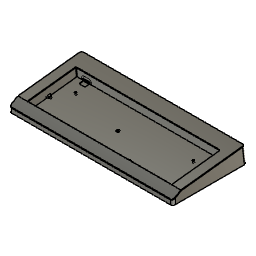
Bezel (Autodesk Fusion 360 design; units mm, degrees)
Autodesk Fusion 360 part; units mm, degrees
note: some values were not read from the file. Set by a fixed rule: which sketch regions a step uses.
sketch "スケッチ1" plane through (0, 0, 0) normal (1, 0, 0) x (0, 1, 0)
  line L0 (17.006428, 19.886797) -> (113.581613, 30.890149)
  line L1 (20.037658, 2.115707) -> (115.61927, 13.005856)
  line L2 (115.61927, 13.005856) -> (113.581613, 30.890149)
  line L3 (20.037658, 2.115707) -> (0.037658, 2.115707)
  line L4 (0.037658, 2.115707) -> (0.037658, 10.089873)
  line L5 (0.037658, 10.089873) -> (17.006428, 19.886797)
  line L6 (113.581613, 30.890149) -> (144.38234, 34.399449)
  line L7 (144.38234, 34.399449) -> (146.419998, 16.515155)
  line L8 (146.419998, 16.515155) -> (139.289315, 0.115707)
  line L9 (0.037658, 2.115707) -> (0.037658, 0.115707)
  line L10 (0.037658, 0.115707) -> (139.000002, 0.115707)
  line L11 (139.000002, 0.115707) -> (139.289315, 0.115707)
  line L12 (115.61927, 13.005856) -> (146.419998, 16.515155)
  line L13 (139.289315, 0.115707) -> (149.000002, 0.115707)
  line L14 (146.419998, 16.515155) -> (148.288479, 0.115707)
  line L15 (0.037658, 10.089873) -> (-9.962342, 4.31637)
  line L16 (0.037658, 0.115707) -> (-9.962342, 0.115707)
  line L17 (-9.962342, 0.115707) -> (-9.962342, 4.31637)
  dimension "d5" = 90
  dimension "d6" = 20
  dimension "d7" = 31
  dimension "d8" = 150
  dimension "d9" = 2
  dimension "d10" = 120
  dimension "d11" = 97.2
  dimension "d152" = 10
  constraint perpendicular L3 L4
  constraint perpendicular L2 L6
  constraint perpendicular L6 L7
  constraint perpendicular L3 L9
  constraint perpendicular L9 L10
  constraint perpendicular L7 L12
  constraint parallel L11 L13
  constraint perpendicular L12 L14
  constraint parallel L5 L15
  constraint perpendicular L9 L16
  constraint perpendicular L16 L17
  measures "d5" angle of L0 L2
  measures "d8" angle of L7 L8
  measures "d10" angle of L4 L5
extrude "押し出し1" add sketch "スケッチ1" along normal blind 316.7 contours L0 L1 L2 L3 L4 L5 | L2 L6 L7 L12 | L1 L3 L8 L9 L10 L11 L12 | L8 L13 L14 picked at (50.208566, 17.630884) picked at (135.473869, 21.30682) picked at (133.679757, 9.878906) picked at (144.665931, 5.58219)
sketch "スケッチ2" plane through (0, -2.018841, 17.719141) normal (0, -0.113203, 0.993572) x (1, 0, 0)
  line L0 (0, 147.348358) -> (0, 19.148358)
  line L1 (0, 19.148358) -> (316.7, 19.148358)
  line L2 (316.7, 19.148358) -> (316.7, 147.348358)
  line L3 (316.7, 147.348358) -> (0, 147.348358)
  line L4 (15.7, 116.348358) -> (301, 116.348358)
  line L5 (301.7, 115.648358) -> (301.7, 20.848358)
  line L6 (301, 20.148358) -> (15.7, 20.148358)
  line L7 (15, 20.848358) -> (15, 115.648358)
  arc A0 (15.7, 116.348358) -> (15, 115.648358) centre (15.7, 115.648358) ccw
  arc A1 (15, 20.848358) -> (15.7, 20.148358) centre (15.7, 20.848358) ccw
  arc A2 (301.7, 115.648358) -> (301, 116.348358) centre (301, 115.648358) ccw
  arc A3 (301, 20.148358) -> (301.7, 20.848358) centre (301, 20.848358) ccw
  point P0 (15, 116.348358)
  point P1 (15, 20.148358)
  dimension "d14" = 15
  dimension "d15" = 31
  dimension "d16" = 96.2
  dimension "d17" = 15
  dimension "d24" = 0.7
  dimension "d25" = 0.7
  dimension "d26" = 0.7
  dimension "d27" = 0.7
  constraint horizontal L4
  constraint vertical L5
  constraint horizontal L6
  constraint vertical L7
  constraint tangent L4 A0
  constraint tangent L7 A0
  constraint tangent L6 A1
  constraint tangent L7 A1
  constraint tangent L4 A2
  constraint tangent L5 A2
  constraint tangent L5 A3
  constraint tangent L6 A3
  measures "d14" distance of L0 L7
  measures "d15" distance of L3 L4
  measures "d17" distance of L2 L5
  measures "d24" radius of A0
  measures "d25" radius of A1
  measures "d26" radius of A2
  measures "d27" radius of A3
extrude "押し出し2" cut sketch "スケッチ2" against normal blind 17.5 contours L4 L5 L6 L7 A0 A1 A2 A3 picked at (205.9, 84.281691)
sketch "スケッチ5" plane through (0, -0.037785, 0.331634) normal (0, -0.113203, 0.993572) x (1, 0, 0)
  arc A0 (15, 20.848358) -> (15.7, 20.148358) centre (15.7, 20.848358) ccw
  line L0 (15.7, 20.148358) -> (301, 20.148358)
  arc A1 (301, 20.148358) -> (301.7, 20.848358) centre (301, 20.848358) ccw
  line L1 (301.7, 20.848358) -> (301.7, 115.648358)
  arc A2 (301.7, 115.648358) -> (301, 116.348358) centre (301, 115.648358) ccw
  line L2 (301, 116.348358) -> (15.7, 116.348358)
  arc A3 (15.7, 116.348358) -> (15, 115.648358) centre (15.7, 115.648358) ccw
  line L3 (15, 115.648358) -> (15, 20.848358)
  circle A4 centre (297.7, 59.248358) radius 2
  circle A5 centre (19, 59.248358) radius 2
  line L4 (297.7, 61.248358) -> (299.2, 61.248358)
  line L5 (297.7, 57.248358) -> (299.167726, 57.267307)
  line L6 (301.7, 54.767515) -> (301.7, 52.300068)
  line L7 (301.7, 63.748358) -> (301.7, 68.000001)
  arc A6 (299.2, 61.248358) -> (301.7, 63.748358) centre (299.2, 63.748358) ccw
  arc A7 (301.7, 54.767515) -> (299.167726, 57.267307) centre (299.2, 54.767515) ccw
  line L8 (18.999289, 61.248358) -> (17.500848, 61.247825)
  line L9 (14.999959, 63.748494) -> (15, 63.900354)
  line L10 (18.997926, 57.248359) -> (17.501562, 57.249911)
  line L11 (14.998969, 54.748872) -> (15, 52.269736)
  arc A8 (14.999959, 63.748494) -> (17.500848, 61.247825) centre (17.499959, 63.747825) ccw
  arc A9 (17.501562, 57.249911) -> (14.998969, 54.748872) centre (17.498969, 54.749912) ccw
  circle A10 centre (275.95, 87.898358) radius 2
  circle A11 centre (41.025, 87.848358) radius 2
  circle A12 centre (206.375, 30.573358) radius 2
  point P0 (14.999289, 61.246935)
  point P1 (14.997928, 57.252507)
  dimension "d28" = 4
  dimension "d29" = 4
  dimension "d30" = 4
  dimension "d31" = 4
  dimension "d32" = 39.1
  dimension "d33" = 39.1
  dimension "d34" = 2.5
  dimension "d35" = 2.5
  dimension "d36" = 4
  dimension "d37" = 4
  dimension "d38" = 2.5
  dimension "d39" = 2.5
  dimension "d40" = 4
  dimension "d41" = 25.75
  dimension "d42" = 28.45
  dimension "d43" = 4
  dimension "d44" = 26.025
  dimension "d45" = 28.5
  dimension "d46" = 4
  dimension "d47" = 95.325
  dimension "d48" = 10.425
  constraint tangent A4 L4
  constraint perpendicular L1 L4
  constraint tangent L4 A6
  constraint tangent L7 A6
  constraint tangent L5 A7
  constraint tangent L6 A7
  constraint tangent A5 L8
  constraint tangent A5 L10
  constraint tangent L8 A8
  constraint tangent L9 A8
  constraint tangent L10 A9
  constraint tangent L11 A9
  measures "d28" diameter of A4
  measures "d30" diameter of A5
  measures "d34" radius of A6
  measures "d35" radius of A7
  measures "d38" radius of A8
  measures "d39" radius of A9
  measures "d40" diameter of A10
  measures "d43" diameter of A11
  measures "d46" diameter of A12
extrude "押し出し4" add sketch "スケッチ5" along normal blind 3.5 contours A4 | L3 A5 L8 L10 A8 A9 | A5 | L1 A4 L4 L5 A6 A7 | A10 | A11 | A12 picked at (297.197858, 59.608279) picked at (16.24367, 59.199293) picked at (18.424304, 58.865784) picked at (300.453653, 59.258571) picked at (275.290779, 87.997719) picked at (41.655264, 87.362598) picked at (206.217662, 29.380725)
sketch "スケッチ6" plane through (0, -0.037785, 0.331634) normal (0, -0.113203, 0.993572) x (1, 0, 0)
  circle A0 centre (275.95, 87.898358) radius 2
  circle A1 centre (41.025, 87.848358) radius 2
  circle A2 centre (206.375, 30.573358) radius 2
  arc A3 (301.7, 54.767515) -> (299.167726, 57.267307) centre (299.2, 54.767515) ccw
  line L0 (299.167726, 57.267307) -> (297.7, 57.248358)
  arc A4 (297.7, 61.248358) -> (297.7, 57.248358) centre (297.7, 59.248358) ccw
  line L1 (297.7, 61.248358) -> (299.2, 61.248358)
  arc A5 (299.2, 61.248358) -> (301.7, 63.748358) centre (299.2, 63.748358) ccw
  line L2 (301.7, 63.748358) -> (301.7, 115.648358)
  arc A6 (301.7, 115.648358) -> (301, 116.348358) centre (301, 115.648358) ccw
  line L3 (301, 116.348358) -> (15.7, 116.348358)
  arc A7 (15.7, 116.348358) -> (15, 115.648358) centre (15.7, 115.648358) ccw
  line L4 (15, 115.648358) -> (15, 63.733545)
  arc A8 (15, 63.733545) -> (17.500848, 61.247825) centre (17.499959, 63.747825) ccw
  line L5 (17.500848, 61.247825) -> (18.999289, 61.248358)
  arc A9 (18.997926, 57.248359) -> (18.999289, 61.248358) centre (19, 59.248358) ccw
  line L6 (18.997926, 57.248359) -> (17.501562, 57.249911)
  arc A10 (17.501562, 57.249911) -> (15, 54.821709) centre (17.498969, 54.749912) ccw
  line L7 (15, 54.821709) -> (15, 20.848358)
  arc A11 (15, 20.848358) -> (15.7, 20.148358) centre (15.7, 20.848358) ccw
  line L8 (15.7, 20.148358) -> (301, 20.148358)
  arc A12 (301, 20.148358) -> (301.7, 20.848358) centre (301, 20.848358) ccw
  circle A13 centre (144.025, 68.748358) radius 0.85
  line L9 (301.7, 20.848358) -> (301.7, 54.767515)
  dimension "d51" = 1.7
  dimension "d52" = 129.025
  dimension "d53" = 48.6
  measures "d51" diameter of A13
extrude "押し出し5" cut sketch "スケッチ6" against normal blind 6 contours A13 picked at (144.088048, 68.472128)
sketch "スケッチ7" plane through (0, 115.600454, 13.171008) normal (0, -0.993572, -0.113203) x (1, 0, 0)
  line L0 (301, 17.833779) -> (15.7, 17.833779)
  line L1 (15.7, 17.833779) -> (15.7, 0.333779)
  line L2 (15.7, 0.333779) -> (301, 0.333779)
  line L3 (301, 0.333779) -> (301, 17.833779)
  line L4 (28, 0.333779) -> (40, 0.333779)
  line L5 (41, 1.333779) -> (41, 3.333779)
  line L6 (40, 4.333779) -> (28, 4.333779)
  line L7 (27, 3.333779) -> (27, 1.333779)
  line L8 (15, 17.833779) -> (15, 0.333779)
  arc A0 (28, 4.333779) -> (27, 3.333779) centre (28, 3.333779) ccw
  arc A1 (27, 1.333779) -> (28, 0.333779) centre (28, 1.333779) ccw
  arc A2 (41, 3.333779) -> (40, 4.333779) centre (40, 3.333779) ccw
  arc A3 (40, 0.333779) -> (41, 1.333779) centre (40, 1.333779) ccw
  point P0 (27, 0.333779)
  point P1 (41, 4.333779)
  point P2 (27, 4.333779)
  dimension "d56" = 4
  dimension "d57" = 12
  dimension "d58" = 14
  dimension "d85" = 1
  dimension "d86" = 1
  dimension "d87" = 1
  dimension "d88" = 1
  constraint horizontal L4
  constraint vertical L5
  constraint horizontal L6
  constraint vertical L7
  constraint tangent L6 A0
  constraint tangent L7 A0
  constraint tangent L4 A1
  constraint tangent L7 A1
  constraint tangent L5 A2
  constraint tangent L6 A2
  constraint tangent L4 A3
  constraint tangent L5 A3
  measures "d57" distance of L7 L8
  measures "d85" radius of A0
  measures "d86" radius of A1
  measures "d87" radius of A2
  measures "d88" radius of A3
extrude "押し出し6" cut sketch "スケッチ7" against normal blind 40 contours L2 L4 L5 L6 L7 A0 A1 A2 A3 picked at (36, 1.667113)
sketch "スケッチ8" plane through (0, 146.401181, 16.680308) normal (0, 0.993572, 0.113203) x (-1, 0, 0)
  line L0 (-41, 1.333779) -> (-41, 3.333779)
  line L1 (-40, 4.333779) -> (-28, 4.333779)
  line L2 (-27, 3.333779) -> (-27, 1.333779)
  line L3 (0, -16.67177) -> (0, 17.833779)
  line L4 (0, 17.833779) -> (-316.7, 17.833779)
  line L5 (-316.7, 17.833779) -> (-316.7, -16.67177)
  circle A0 centre (-34, 1.833779) radius 10
  line L6 (-38.586053, 8.833779) -> (-29.417172, 8.833779)
  line L7 (-26.858572, 8.833779) -> (-26.858572, -5.166221)
  line L8 (-29.417172, -5.166221) -> (-38.586053, -5.166221)
  line L9 (-41.141428, -5.166221) -> (-41.141428, 8.833779)
  line L10 (-28, 0.333779) -> (-40, 0.333779)
  line L11 (-316.7, -16.67177) -> (0, -16.67177)
  arc A1 (-40, 4.333779) -> (-41, 3.333779) centre (-40, 3.333779) ccw
  arc A2 (-27, 3.333779) -> (-28, 4.333779) centre (-28, 3.333779) ccw
  arc A3 (-28, 0.333779) -> (-27, 1.333779) centre (-28, 1.333779) ccw
  arc A4 (-41, 1.333779) -> (-40, 0.333779) centre (-40, 1.333779) ccw
  arc A5 (-43.166662, 5.838281) -> (-43.166662, -2.170722) centre (-34.015731, 1.833779) ccw
  arc A6 (-24.834739, -2.166547) -> (-24.834739, 5.834106) centre (-33.998857, 1.833779) ccw
  arc A7 (-38.586053, 8.833779) -> (-43.166662, 5.838281) centre (-38.586053, 3.833779) ccw
  arc A8 (-24.834739, 5.834106) -> (-29.417172, 8.833779) centre (-29.417172, 3.833779) ccw
  arc A9 (-43.166662, -2.170722) -> (-38.586053, -5.166221) centre (-38.586053, -0.166221) ccw
  arc A10 (-29.417172, -5.166221) -> (-24.834739, -2.166547) centre (-29.417172, -0.166221) ccw
  dimension "d61" = 20
  dimension "d62" = 34
  dimension "d65" = 14
  dimension "d156" = 14
  dimension "d157" = 5
  dimension "d158" = 5
  dimension "d159" = 5
  dimension "d160" = 5
  dimension "d161" = 14.5
  dimension "d162" = 2
  dimension "d163" = 16
  constraint horizontal L6
  constraint vertical L7
  constraint horizontal L8
  constraint vertical L9
  constraint tangent L6 A7
  constraint tangent A5 A7
  constraint tangent L6 A8
  constraint tangent A6 A8
  constraint tangent A5 A9
  constraint tangent L8 A9
  constraint tangent L8 A10
  constraint tangent A6 A10
  measures "d61" diameter of A0
  measures "d157" radius of A7
  measures "d158" radius of A8
  measures "d159" radius of A9
  measures "d160" radius of A10
extrude "押し出し7" cut sketch "スケッチ8" against normal blind 30 contours L0 L1 L2 L10 A1 A2 A3 A4 | A0 L7 A6 A8 A10 | L6 L7 L8 L9 A7 A8 A9 A10 | A0 L9 A7 A9 | A0 A5 A7 A9 picked at (-36, 3.000446) picked at (-25.905714, 1.833779) picked at (-32.472391, -1.499554) picked at (-42.094286, 1.833779) picked at (-43.120762, -2.270015)
sketch "スケッチ10" plane through (0, -0.037785, 0.331634) normal (0, -0.113203, 0.993572) x (1, 0, 0)
  line L0 (40, 117.348358) -> (28, 117.348358)
  line L1 (28, 116.348358) -> (15.7, 116.348358)
  arc A0 (15.7, 116.348358) -> (15, 115.648358) centre (15.7, 115.648358) ccw
  line L2 (15, 115.648358) -> (15, 63.733545)
  arc A1 (15, 63.733545) -> (17.500848, 61.247825) centre (17.499959, 63.747825) ccw
  line L3 (17.500848, 61.247825) -> (18.999289, 61.248358)
  arc A2 (18.997926, 57.248359) -> (18.999289, 61.248358) centre (19, 59.248358) ccw
  line L4 (18.997926, 57.248359) -> (17.501562, 57.249911)
  arc A3 (17.501562, 57.249911) -> (15, 54.821709) centre (17.498969, 54.749912) ccw
  line L5 (15, 54.821709) -> (15, 20.848358)
  arc A4 (15, 20.848358) -> (15.7, 20.148358) centre (15.7, 20.848358) ccw
  line L6 (15.7, 20.148358) -> (301, 20.148358)
  arc A5 (301, 20.148358) -> (301.7, 20.848358) centre (301, 20.848358) ccw
  line L7 (301.7, 20.848358) -> (301.7, 54.767515)
  arc A6 (301.7, 54.767515) -> (299.167726, 57.267307) centre (299.2, 54.767515) ccw
  line L8 (299.167726, 57.267307) -> (297.7, 57.248358)
  arc A7 (297.7, 61.248358) -> (297.7, 57.248358) centre (297.7, 59.248358) ccw
  line L9 (297.7, 61.248358) -> (299.2, 61.248358)
  arc A8 (299.2, 61.248358) -> (301.7, 63.748358) centre (299.2, 63.748358) ccw
  line L10 (301.7, 63.748358) -> (301.7, 115.648358)
  arc A9 (301.7, 115.648358) -> (301, 116.348358) centre (301, 115.648358) ccw
  circle A10 centre (206.375, 30.573358) radius 2
  circle A11 centre (41.025, 87.848358) radius 2
  circle A12 centre (275.95, 87.898358) radius 2
  circle A13 centre (144.025, 68.748358) radius 0.85
  line L11 (29, 116.348358) -> (39, 116.348358)
  line L12 (40, 115.348358) -> (40, 108.348358)
  line L13 (39, 107.348358) -> (29, 107.348358)
  line L14 (28, 107.348358) -> (28, 115.348358)
  line L15 (40, 117.348358) -> (28, 117.348358)
  line L16 (28, 117.348358) -> (28, 108.348358)
  line L17 (28, 107.348358) -> (39, 107.348358)
  line L18 (40, 108.348358) -> (40, 115.348358)
  arc A14 (40, 115.348358) -> (39, 116.348358) centre (39, 115.348358) ccw
  arc A15 (39, 107.348358) -> (40, 108.348358) centre (39, 108.348358) ccw
  arc A16 (29, 116.348358) -> (28, 115.348358) centre (29, 115.348358) ccw
  arc A17 (28, 108.348358) -> (29, 107.348358) centre (29, 108.348358) ccw
  line L19 (28, 117.348358) -> (28, 116.348358)
  line L20 (301, 116.348358) -> (40, 116.348358)
  line L21 (40, 116.348358) -> (40, 117.348358)
  arc A18 (39, 107.348358) -> (40, 108.348358) centre (39, 108.348358) ccw
  arc A19 (40, 115.348358) -> (39, 116.348358) centre (39, 115.348358) ccw
  point P0 (28, 116.348358)
  point P1 (40, 116.348358)
  dimension "d73" = 12
  dimension "d74" = 9
  dimension "d77" = 1
  dimension "d78" = 1
  dimension "d79" = 1
  dimension "d80" = 1
  dimension "d89" = 1
  dimension "d90" = 1
  constraint horizontal L11
  constraint vertical L12
  constraint horizontal L13
  constraint vertical L14
  constraint horizontal L15
  constraint vertical L16
  constraint horizontal L17
  constraint vertical L18
  constraint tangent L11 A14
  constraint tangent L12 A14
  constraint tangent L12 A15
  constraint tangent L13 A15
  constraint tangent L11 A16
  constraint tangent L14 A16
  constraint tangent L13 A17
  constraint tangent L16 A17
  constraint tangent L17 A18
  constraint tangent L18 A18
  constraint tangent L18 A19
  constraint tangent L11 A19
  measures "d77" radius of A14
  measures "d78" radius of A15
  measures "d79" radius of A16
  measures "d80" radius of A17
  measures "d89" radius of A18
  measures "d90" radius of A19
extrude "押し出し8" cut sketch "スケッチ10" against normal blind 1 contours L11 L12 L13 L14 L16 L17 L18 A14 A15 A16 A17 A18 A19 picked at (35.666667, 110.348358)
chamfer "面取り2" distance 0.75 angle 45 8 edges at (158.35, 113.581613, 30.890149) (301.494975, 113.377905, 30.86694) (301.7, 65.790806, 25.445075) (301.494975, 18.203707, 20.02321) (158.35, 18, 20) (15.205025, 18.203707, 20.02321) (15, 65.790806, 25.445075) (15.205025, 113.377905, 30.86694)
chamfer "面取り3" distance 0.75 angle 45 8 edges at (24, 146.193591, 18.502299) (34.001613, 146.986014, 11.547296) (44, 146.193591, 18.502299) (34.001613, 145.401169, 25.457302) (26.707032, 146.895655, 12.340363) (41.218787, 146.901194, 12.291749) (41.218787, 145.485989, 24.712849) (26.707032, 145.491527, 24.664235)
sketch "スケッチ12" plane through (0, 146.401181, 16.680308) normal (0, 0.993572, 0.113203) x (-1, 0, 0)
  line L0 (-10, -13.92177) -> (-306.7, -13.92177)
  line L1 (-309.7, -10.92177) -> (-309.7, 12.083779)
  line L2 (-306.7, 15.083779) -> (-10, 15.083779)
  line L3 (-7, 12.083779) -> (-7, -10.92177)
  arc A0 (-306.7, 15.083779) -> (-309.7, 12.083779) centre (-306.7, 12.083779) ccw
  arc A1 (-309.7, -10.92177) -> (-306.7, -13.92177) centre (-306.7, -10.92177) ccw
  arc A2 (-10, -13.92177) -> (-7, -10.92177) centre (-10, -10.92177) ccw
  arc A3 (-7, 12.083779) -> (-10, 15.083779) centre (-10, 12.083779) ccw
  line L4 (-316.7, -16.67177) -> (0, -16.67177)
  line L5 (0, 17.833779) -> (-316.7, 17.833779)
  line L6 (-316.7, 17.833779) -> (-316.7, -16.67177)
  line L7 (0, -16.67177) -> (0, 17.833779)
  arc A4 (-24.177884, -2.535263) -> (-24.177884, 6.202822) centre (-34, 1.833779) ccw
  arc A5 (-29.417172, -5.916221) -> (-24.177884, -2.535263) centre (-29.417172, -0.166221) ccw
  line L8 (-29.417172, -5.916221) -> (-38.586053, -5.916221)
  arc A6 (-43.738216, -2.719203) -> (-38.586053, -5.916221) centre (-38.586053, -0.166221) ccw
  arc A7 (-43.738216, 6.386761) -> (-43.738216, -2.719203) centre (-34, 1.833779) ccw
  arc A8 (-38.586053, 9.583779) -> (-43.738216, 6.386761) centre (-38.586053, 3.833779) ccw
  line L9 (-38.586053, 9.583779) -> (-29.417172, 9.583779)
  arc A9 (-24.177884, 6.202821) -> (-29.417172, 9.583779) centre (-29.417172, 3.833779) ccw
  dimension "d100" = 3
  dimension "d101" = 3
  dimension "d102" = 3
  dimension "d103" = 3
  constraint horizontal L0
  constraint vertical L1
  constraint horizontal L2
  constraint vertical L3
  constraint tangent L1 A0
  constraint tangent L2 A0
  constraint tangent L0 A1
  constraint tangent L1 A1
  constraint tangent L0 A2
  constraint tangent L3 A2
  constraint tangent L2 A3
  constraint tangent L3 A3
  measures "d100" radius of A0
  measures "d101" radius of A1
  measures "d102" radius of A2
  measures "d103" radius of A3
extrude "押し出し9" cut sketch "スケッチ12" against normal blind 2.5 contours L0 L1 L2 L3 A0 A1 A2 A3 | A4 A5 L8 A6 A7 A8 L9 A9 picked at (-219.383333, 0.998596) picked at (-32.473466, -0.749554)
sketch "スケッチ13" plane through (0, 143.917252, 16.3973) normal (0, 0.993572, 0.113203) x (-1, 0, 0)
  arc A0 (-10, -13.92177) -> (-7, -10.92177) centre (-10, -10.92177) ccw
  line L0 (-7, -10.92177) -> (-7, 12.083779)
  arc A1 (-7, 12.083779) -> (-10, 15.083779) centre (-10, 12.083779) ccw
  line L1 (-10, 15.083779) -> (-306.7, 15.083779)
  arc A2 (-306.7, 15.083779) -> (-309.7, 12.083779) centre (-306.7, 12.083779) ccw
  line L2 (-309.7, 12.083779) -> (-309.7, -10.92177)
  arc A3 (-309.7, -10.92177) -> (-306.7, -13.92177) centre (-306.7, -10.92177) ccw
  line L3 (-306.7, -13.92177) -> (-10, -13.92177)
  circle A4 centre (-300.7, 1.583779) radius 1.35
  circle A5 centre (-16, 1.583779) radius 1.35
  circle A6 centre (-52, 1.583779) radius 1.35
  line L4 (-29.417172, -5.166221) -> (-38.586053, -5.166221)
  arc A7 (-43.062471, -2.393705) -> (-38.586053, -5.166221) centre (-38.586053, -0.166221) ccw
  arc A8 (-43.062471, 6.061264) -> (-43.062471, -2.393705) centre (-34, 1.833779) ccw
  arc A9 (-38.586053, 8.833779) -> (-43.062471, 6.061264) centre (-38.586053, 3.833779) ccw
  line L5 (-38.586053, 8.833779) -> (-29.417172, 8.833779)
  arc A10 (-24.862184, 5.895837) -> (-29.417172, 8.833779) centre (-29.417172, 3.833779) ccw
  arc A11 (-24.862184, -2.228278) -> (-24.862184, 5.895837) centre (-34, 1.833779) ccw
  arc A12 (-29.417172, -5.166221) -> (-24.862184, -2.228278) centre (-29.417172, -0.166221) ccw
  dimension "d104" = 2.7
  dimension "d105" = 2.7
  dimension "d107" = 9
  dimension "d108" = 2.7
  dimension "d111" = 13.5
  dimension "d112" = 15.505549
  dimension "d113" = 13.5
  dimension "d114" = 13.5
  dimension "d166" = 18
  dimension "d167" = 18
  dimension "d168" = 9
  measures "d104" diameter of A4
  measures "d105" diameter of A5
  measures "d108" diameter of A6
extrude "押し出し10" cut sketch "スケッチ13" against normal blind 4 contours A4 | A5 | A6 picked at (-301.029873, 1.277702) picked at (-16.035865, 2.002672) picked at (-51.555026, 1.907206)
sketch "スケッチ14" plane through (0, -0.433996, 3.809135) normal (0, -0.113203, 0.993572) x (1, 0, 0)
  circle A0 centre (41.025, 87.848358) radius 2
  circle A1 centre (41.025, 87.848358) radius 0.85
  circle A2 centre (19, 59.248358) radius 0.85
  circle A3 centre (206.375, 30.573358) radius 0.85
  circle A4 centre (297.7, 59.248358) radius 0.85
  line L0 (301, 20.148358) -> (15.7, 20.148358)
  line L1 (15, 20.848358) -> (15, 115.648358)
  line L2 (301.7, 115.648358) -> (301.7, 20.848358)
  line L3 (15.7, 116.348358) -> (301, 116.348358)
  circle A5 centre (206.375, 30.573358) radius 2
  circle A6 centre (275.95, 87.898358) radius 0.85
  circle A7 centre (275.95, 87.898358) radius 2
  dimension "d117" = 1.7
  dimension "d118" = 1.7
  dimension "d119" = 1.7
  dimension "d121" = 1.7
  dimension "d122" = 39.1
  dimension "d123" = 4
  dimension "d124" = 39.1
  dimension "d125" = 4
  dimension "d165" = 1.7
  constraint concentric A0 A1
  measures "d117" diameter of A1
  measures "d118" diameter of A2
  measures "d119" diameter of A3
  measures "d121" diameter of A4
  measures "d165" diameter of A6
extrude "押し出し11" cut sketch "スケッチ14" against normal blind 4 contours A1 | A2 | A3 | A4 | A6 picked at (41.358793, 88.041073) picked at (19.063048, 58.972128) picked at (206.837301, 30.696291) picked at (297.934101, 59.407965) picked at (275.742302, 87.705642)
sketch "スケッチ15" plane through (0, 0, 0.115707) normal (0, 0, -1) x (1, 0, 0)
  circle A0 centre (10, -10.037658) radius 3.75
  circle A1 centre (306.7, -10.037658) radius 3.75
  circle A2 centre (306.7, -138.288479) radius 3.75
  circle A3 centre (10, -138.288479) radius 3.75
  line L0 (316.7, -148.288479) -> (316.7, -0.037658)
  line L1 (0, -0.037658) -> (0, -148.288479)
  line L2 (0, -148.288479) -> (316.7, -148.288479)
  line L3 (316.7, -0.037658) -> (0, -0.037658)
  dimension "d133" = 7.5
  dimension "d136" = 7.5
  dimension "d139" = 7.5
  dimension "d142" = 7.5
  dimension "d172" = 10
  dimension "d173" = 10
  dimension "d174" = 10
  dimension "d175" = 10
  dimension "d176" = 10
  dimension "d177" = 10
  dimension "d178" = 10
  dimension "d179" = 10
  measures "d133" diameter of A0
  measures "d136" diameter of A1
  measures "d139" diameter of A2
  measures "d142" diameter of A3
extrude "押し出し12" cut sketch "スケッチ15" against normal blind 0.5 contours A0 | A1 | A2 | A3 picked at (11.101053, -10.915719) picked at (307.826211, -10.580013) picked at (307.003309, -139.227123) picked at (9.083685, -137.438263)
extrude "押し出し13" add 1 faces at (316.7, 103.225749, 18.133984) along direction (1, 0, 0) blind 5
extrude "押し出し14" add 1 faces at (0, 103.225749, 18.133984) along direction (-1, 0, 0) blind 5
fillet "フィレット3" radius 5 4 edges at (321.7, 0.037658, 5.10279) (-5, 0.037658, 5.10279) (321.7, 146.33541, 17.257578) (-5, 146.33541, 17.257578)
chamfer "面取り4" distance 0.75 angle 45 18 edges at (158.35, 0.037658, 10.089873) (320.235534, 1.502124, 10.935383) (321.7, 11.022043, 16.43171) (-5, 11.022043, 16.43171) (-3.535534, 1.502124, 10.935383) (321.7, 78.210454, 26.860115) (-5, 78.210454, 26.860115) (-3.535534, 142.927288, 34.233667) (158.35, 144.38234, 34.399449) (320.235534, 142.927288, 34.233667) (321.7, 74.146894, 0.115707) (320.235534, 146.814538, 0.115707) (158.35, 148.288479, 0.115707) (-3.535534, 146.814538, 0.115707) (-5, 74.146894, 0.115707) (-3.535534, 1.502124, 0.115707) (158.35, 0.037658, 0.115707) (320.235534, 1.502124, 0.115707)
chamfer "面取り5" distance 0.75 angle 45 8 edges at (44, 143.709662, 18.219291) (41.218787, 143.002059, 24.429841) (26.707032, 143.007598, 24.381227) (34.001613, 142.917239, 25.174294) (41.218787, 144.417265, 12.008741) (34.001613, 144.502084, 11.264288) (26.707032, 144.411726, 12.057355) (24, 143.709662, 18.219291)
sketch "スケッチ19" plane through (0, -0.037785, 0.331634) normal (0, -0.113203, 0.993572) x (1, 0, 0)
  line L0 (39, 107.348358) -> (29, 107.348358)
  arc A0 (28, 108.348358) -> (29, 107.348358) centre (29, 108.348358) ccw
  line L1 (28, 108.348358) -> (28, 115.348358)
  arc A1 (29, 116.348358) -> (28, 115.348358) centre (29, 115.348358) ccw
  line L2 (29, 116.348358) -> (39, 116.348358)
  line L3 (40, 115.348358) -> (40, 108.348358)
  line L4 (40, 117.348358) -> (28, 117.348358)
  line L5 (28, 117.348358) -> (28, 116.348358)
  line L6 (28, 116.348358) -> (15.7, 116.348358)
  arc A2 (15.7, 116.348358) -> (15, 115.648358) centre (15.7, 115.648358) ccw
  line L7 (15, 115.648358) -> (15, 63.733545)
  arc A3 (15, 63.733545) -> (17.500848, 61.247825) centre (17.499959, 63.747825) ccw
  line L8 (17.500848, 61.247825) -> (18.999289, 61.248358)
  arc A4 (18.997926, 57.248359) -> (18.999289, 61.248358) centre (19, 59.248358) ccw
  line L9 (18.997926, 57.248359) -> (17.501562, 57.249911)
  arc A5 (17.501562, 57.249911) -> (15, 54.821709) centre (17.498969, 54.749912) ccw
  line L10 (15, 54.821709) -> (15, 20.848358)
  arc A6 (15, 20.848358) -> (15.7, 20.148358) centre (15.7, 20.848358) ccw
  line L11 (15.7, 20.148358) -> (301, 20.148358)
  arc A7 (301, 20.148358) -> (301.7, 20.848358) centre (301, 20.848358) ccw
  line L12 (301.7, 20.848358) -> (301.7, 54.767515)
  arc A8 (301.7, 54.767515) -> (299.167726, 57.267307) centre (299.2, 54.767515) ccw
  line L13 (299.167726, 57.267307) -> (297.7, 57.248358)
  arc A9 (297.7, 61.248358) -> (297.7, 57.248358) centre (297.7, 59.248358) ccw
  line L14 (297.7, 61.248358) -> (299.2, 61.248358)
  arc A10 (299.2, 61.248358) -> (301.7, 63.748358) centre (299.2, 63.748358) ccw
  line L15 (301.7, 63.748358) -> (301.7, 115.648358)
  arc A11 (301.7, 115.648358) -> (301, 116.348358) centre (301, 115.648358) ccw
  line L16 (301, 116.348358) -> (40, 116.348358)
  line L17 (40, 116.348358) -> (40, 117.348358)
  circle A12 centre (144.025, 68.748358) radius 0.85
  circle A13 centre (275.95, 87.898358) radius 2
  circle A14 centre (41.025, 87.848358) radius 2
  circle A15 centre (206.375, 30.573358) radius 2
  arc A16 (39, 107.348358) -> (40, 108.348358) centre (39, 108.348358) ccw
  arc A17 (40, 115.348358) -> (39, 116.348358) centre (39, 115.348358) ccw
  circle A18 centre (144.025, 68.748358) radius 3
  dimension "d169" = 6
  constraint concentric A12 A18
  measures "d169" diameter of A18
extrude "押し出し15" cut sketch "スケッチ19" against normal blind 0.5 contours A18 picked at (142.46076, 70.403078)
equation "d11 = 96.20 mm + 1 mm"
equation "d32 = 38.6 mm + 0.5 mm"
equation "d33 = 38.6 mm + 0.5 mm"
equation "d41 = 25.45 mm + 0.3 mm"
equation "d42 = 28.4 mm + 0.05 mm"
equation "d44 = 25.7 mm + 0.325 mm"
equation "d47 = 95 mm + 0.325 mm"
equation "d48 = 9.9 mm + 0.525 mm"
equation "d52 = 128.7 mm + 0.325 mm"
equation "d53 = 47.5 mm + 1.1 mm"
equation "d62 = 12.5 mm + 6 mm + 15.5 mm"
equation "d122 = 38.6 mm + 0.5 mm"
equation "d124 = 38.6 mm + 0.5 mm"
